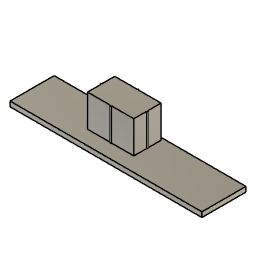
Curtains Cap Opposite (Autodesk Fusion 360 design; units mm, degrees)
Autodesk Fusion 360 part; units mm, degrees
sketch "Sketch1" plane through (0, 0, 0) normal (0, 0, 1) x (1, 0, 0)
  line L0 (77.5, 0) -> (77.5, 17.8)
  line L1 (0, 17.8) -> (0, 0)
  line L2 (44.2, 5.8) -> (44.2, 16.8)
  line L3 (44.2, 16.8) -> (25.5, 16.8)
  line L4 (25.5, 16.8) -> (25.5, 5.8)
  line L5 (77.5, 17.8) -> (62.1, 17.8)
  line L6 (58.4, 17.8) -> (26.9, 17.8)
  line L7 (23.2, 17.8) -> (0, 17.8)
  line L8 (0, 0) -> (39.3, 0)
  line L9 (46, 0) -> (77.5, 0)
  line L10 (25.5, 5.8) -> (31.5, 5.8)
  line L11 (38.2, 5.8) -> (44.2, 5.8)
  line L12 (31.5, 5.8) -> (38.2, 5.8)
  line L13 (39.3, 0) -> (46, 0)
  line L14 (62.1, 17.8) -> (58.4, 17.8)
  line L15 (23.2, 17.8) -> (26.9, 17.8)
  circle A0 centre (34.85, 5.8) radius 0.3
  circle A1 centre (25.5, 11.3) radius 0.3
  circle A2 centre (44.2, 11.3) radius 0.3
  circle A3 centre (34.85, 16.8) radius 0.3
  dimension "d1" = 77.5
  dimension "d2" = 17.8
  dimension "d25" = 11
  dimension "d26" = 1
  dimension "d44" = 25.5
  dimension "d45" = 18.7
  dimension "d46" = 0.6
  dimension "d47" = 0.6
  dimension "d48" = 0.6
  dimension "d49" = 0.6
  constraint horizontal L8
  constraint vertical L0
  constraint horizontal L5
  constraint vertical L1
  constraint coincident L1.end L8.start
  constraint coincident L6.start L5
  constraint coincident L7.start L5
  constraint coincident L6.end L5
  constraint horizontal L10
  constraint vertical L2
  constraint horizontal L3
  constraint vertical L4
  constraint collinear L5 L6
  constraint collinear L6 L7
  constraint coincident L11.start L10
  constraint coincident L9.start L8
  constraint collinear L8 L9
  constraint collinear L10 L11
  constraint horizontal L15
  constraint midpoint L12 A0.centre
  constraint midpoint L4 A1.centre
  constraint midpoint L2 A2.centre
  constraint midpoint L3 A3.centre
  measures "d1" distance of L1.end L0.start
  measures "d2" distance of L1.end L1.start
  measures "d25" distance of L3 L10
  measures "d26" distance of L3 L5
  measures "d44" distance of L1 L4
  measures "d45" distance of L2.end L3.end
  measures "d46" diameter of A0
  measures "d47" diameter of A1
  measures "d48" diameter of A2
  measures "d49" diameter of A3
extrude "Extrude1" add sketch "Sketch1" along normal blind 2 contours L0 L1 L5 L6 L7 L8 L9 L13 L14 L15 | L2 A2 | L12 A0 | L3 A3 | L4 A1 picked at (44.4269, 11.2718) picked at (34.8425, 5.7003) picked at (34.8723, 16.8975) picked at (25.4025, 11.3223)
extrude "Extrude2" add sketch "Sketch1" along normal blind 15 contours L2 L3 L4 L10 L11 L12 A0 A1 A2 A3 | L2 A2 | L2 A2 | L12 A0 | L12 A0 | L3 A3 | L3 A3 | L4 A1 | L4 A1
sketch "Sketch2" plane through (0, 0, 0) normal (0, 0, 1) x (1, 0, 0)
  line L0 (25.5, 5.8) -> (31.5, 5.8)
  line L1 (31.5, 5.8) -> (38.2, 5.8)
  line L2 (38.2, 5.8) -> (44.2, 5.8)
  line L3 (44.2, 5.8) -> (44.2, 16.8)
  line L4 (25.5, 16.8) -> (25.5, 5.8)
  line L5 (44.2, 16.8) -> (25.5, 16.8)
  line L6 (48, 8) -> (37.3, 8)
  line L7 (37.3, 8) -> (37.3, 14.6)
  line L8 (37.3, 14.6) -> (48, 14.6)
  line L9 (48, 14.6) -> (48, 8)
  line L10 (48, 8) -> (37.3, 14.6) construction
  line L11 (37.3, 8) -> (48, 14.6) construction
  point P0 (42.65, 11.3)
  constraint horizontal L6
  constraint perpendicular L6 L7
  constraint parallel L6 L8
  constraint parallel L7 L9
  constraint coincident L10 P0
  constraint coincident L11 P0
